Autodesk Fusion 360 part; units mm, degrees
(part 3 of 5)
  spline S11 degree 5 poles (-26.6259, 4.9636) (-26.6188, 4.9697) (-26.6047, 4.9821) (-26.5837, 5.0007) (-26.5558, 5.0255) (-26.5211, 5.0567) (-26.4867, 5.0881) (-26.4526, 5.1196) (-26.4187, 5.1512) (-26.385, 5.183) (-26.3516, 5.2149) (-26.3185, 5.2469) (-26.2856, 5.2791) (-26.2529, 5.3114) (-26.2205, 5.3438) (-26.1884, 5.3764) (-26.1566, 5.4091) (-26.125, 5.4419) (-26.0937, 5.4749) (-26.0626, 5.5079) (-26.0318, 5.5412) (-26.0013, 5.5745) (-25.9711, 5.608) (-25.9412, 5.6416) (-25.9115, 5.6753) (-25.8821, 5.7092) (-25.853, 5.7432) (-25.8242, 5.7773) (-25.7957, 5.8115) (-25.7675, 5.8458) (-25.7396, 5.8803) (-25.712, 5.9149) (-25.6847, 5.9496) (-25.6577, 5.9845) (-25.631, 6.0194) (-25.6046, 6.0545) (-25.5785, 6.0897) (-25.5528, 6.125) (-25.5273, 6.1604) (-25.5022, 6.196) (-25.4775, 6.2316) (-25.453, 6.2674) (-25.4289, 6.3033) (-25.4052, 6.3393) (-25.3818, 6.3754) (-25.3588, 6.4117) (-25.3361, 6.448) (-25.3138, 6.4845) (-25.2919, 6.521) (-25.2703, 6.5577) (-25.2491, 6.5945) (-25.2283, 6.6314) (-25.208, 6.6684) (-25.1881, 6.7055) (-25.1686, 6.7428) (-25.1495, 6.7801) (-25.1308, 6.8176) (-25.1125, 6.8552) (-25.0946, 6.8928) (-25.0772, 6.9306) (-25.0603, 6.9685) (-25.044, 7.0065) (-25.0285, 7.0447) (-25.0136, 7.083) (-24.9994, 7.1214) (-24.9856, 7.16) (-24.9721, 7.1986) (-24.959, 7.2372) (-24.9464, 7.2759) (-24.9347, 7.3148) (-24.9243, 7.3539) (-24.9176, 7.3854) (-24.9137, 7.4093) (-24.9115, 7.4253) (-24.9106, 7.4333) knots -1 -1 -1 -1 -1 -1 -0.98571429 -0.97142857 -0.95714286 -0.94285714 -0.92857143 -0.91428571 -0.9 -0.88571429 -0.87142857 -0.85714286 -0.84285714 -0.82857143 -0.81428571 -0.8 -0.78571429 -0.77142857 -0.75714286 -0.74285714 -0.72857143 -0.71428571 -0.7 -0.68571429 -0.67142857 -0.65714286 -0.64285714 -0.62857143 -0.61428571 -0.6 -0.58571429 -0.57142857 -0.55714286 -0.54285714 -0.52857143 -0.51428571 -0.5 -0.48571429 -0.47142857 -0.45714286 -0.44285714 -0.42857143 -0.41428571 -0.4 -0.38571429 -0.37142857 -0.35714286 -0.34285714 -0.32857143 -0.31428571 -0.3 -0.28571429 -0.27142857 -0.25714286 -0.24285714 -0.22857143 -0.21428571 -0.2 -0.18571429 -0.17142857 -0.15714286 -0.14285714 -0.12857143 -0.11428571 -0.1 -0.08571429 -0.07142857 -0.05714286 -0.04285714 -0.02857143 -0.01428571 0 0 0 0 0 0
  line L11 (-24.9106, 7.4333) -> (-24.8202, 8.2036)
  arc A23 (-23.806, 9.0868) -> (-24.8202, 8.2036) centre (-23.827, 8.087) ccw
  arc A24 (-23.806, 9.0868) -> (-23.405, 9.0868) centre (-23.6055, 18.6339) ccw
  arc A25 (-22.3908, 8.2036) -> (-23.405, 9.0868) centre (-23.384, 8.087) ccw
  line L12 (-22.3908, 8.2036) -> (-22.3005, 7.4333)
  spline S12 degree 5 poles (-22.3005, 7.4333) (-22.2995, 7.4253) (-22.2974, 7.4093) (-22.2934, 7.3854) (-22.2867, 7.3539) (-22.2764, 7.3148) (-22.2646, 7.2759) (-22.252, 7.2372) (-22.2389, 7.1986) (-22.2255, 7.16) (-22.2117, 7.1214) (-22.1974, 7.083) (-22.1825, 7.0447) (-22.167, 7.0065) (-22.1507, 6.9685) (-22.1339, 6.9306) (-22.1164, 6.8928) (-22.0985, 6.8552) (-22.0802, 6.8176) (-22.0615, 6.7801) (-22.0425, 6.7428) (-22.023, 6.7055) (-22.0031, 6.6684) (-21.9827, 6.6314) (-21.962, 6.5945) (-21.9408, 6.5577) (-21.9192, 6.521) (-21.8972, 6.4845) (-21.8749, 6.448) (-21.8522, 6.4117) (-21.8292, 6.3754) (-21.8058, 6.3393) (-21.7821, 6.3033) (-21.758, 6.2674) (-21.7336, 6.2316) (-21.7088, 6.196) (-21.6837, 6.1604) (-21.6583, 6.125) (-21.6325, 6.0897) (-21.6065, 6.0545) (-21.5801, 6.0194) (-21.5534, 5.9845) (-21.5264, 5.9496) (-21.4991, 5.9149) (-21.4714, 5.8803) (-21.4435, 5.8458) (-21.4153, 5.8115) (-21.3868, 5.7773) (-21.358, 5.7432) (-21.3289, 5.7092) (-21.2995, 5.6753) (-21.2699, 5.6416) (-21.2399, 5.608) (-21.2097, 5.5745) (-21.1792, 5.5412) (-21.1484, 5.5079) (-21.1174, 5.4749) (-21.0861, 5.4419) (-21.0545, 5.4091) (-21.0226, 5.3764) (-20.9905, 5.3438) (-20.9581, 5.3114) (-20.9255, 5.2791) (-20.8926, 5.2469) (-20.8594, 5.2149) (-20.826, 5.183) (-20.7924, 5.1512) (-20.7585, 5.1196) (-20.7243, 5.0881) (-20.6899, 5.0567) (-20.6553, 5.0255) (-20.6273, 5.0007) (-20.6063, 4.9821) (-20.5922, 4.9697) (-20.5852, 4.9636) knots 0 0 0 0 0 0 0.01428571 0.02857143 0.04285714 0.05714286 0.07142857 0.08571429 0.1 0.11428571 0.12857143 0.14285714 0.15714286 0.17142857 0.18571429 0.2 0.21428571 0.22857143 0.24285714 0.25714286 0.27142857 0.28571429 0.3 0.31428571 0.32857143 0.34285714 0.35714286 0.37142857 0.38571429 0.4 0.41428571 0.42857143 0.44285714 0.45714286 0.47142857 0.48571429 0.5 0.51428571 0.52857143 0.54285714 0.55714286 0.57142857 0.58571429 0.6 0.61428571 0.62857143 0.64285714 0.65714286 0.67142857 0.68571429 0.7 0.71428571 0.72857143 0.74285714 0.75714286 0.77142857 0.78571429 0.8 0.81428571 0.82857143 0.84285714 0.85714286 0.87142857 0.88571429 0.9 0.91428571 0.92857143 0.94285714 0.95714286 0.97142857 0.98571429 1 1 1 1 1 1
  arc A26 (-20.5852, 4.9636) -> (-19.3861, 5.2849) centre (-23.6055, 18.6339) ccw
  spline S13 degree 5 poles (-19.3861, 5.2849) (-19.383, 5.2937) (-19.377, 5.3115) (-19.3681, 5.3381) (-19.3564, 5.3736) (-19.3419, 5.4179) (-19.3278, 5.4623) (-19.314, 5.5066) (-19.3004, 5.551) (-19.2872, 5.5953) (-19.2742, 5.6396) (-19.2615, 5.6839) (-19.2491, 5.7282) (-19.237, 5.7725) (-19.2252, 5.8168) (-19.2136, 5.8611) (-19.2024, 5.9053) (-19.1915, 5.9496) (-19.1808, 5.9938) (-19.1705, 6.0379) (-19.1604, 6.0821) (-19.1507, 6.1262) (-19.1413, 6.1703) (-19.1321, 6.2144) (-19.1233, 6.2584) (-19.1148, 6.3025) (-19.1066, 6.3464) (-19.0987, 6.3904) (-19.0911, 6.4343) (-19.0838, 6.4781) (-19.0769, 6.5219) (-19.0703, 6.5657) (-19.064, 6.6094) (-19.058, 6.6531) (-19.0524, 6.6967) (-19.0471, 6.7403) (-19.0421, 6.7838) (-19.0374, 6.8273) (-19.0331, 6.8706) (-19.0292, 6.914) (-19.0255, 6.9572) (-19.0223, 7.0004) (-19.0194, 7.0436) (-19.0168, 7.0866) (-19.0146, 7.1296) (-19.0128, 7.1725) (-19.0113, 7.2153) (-19.0102, 7.258) (-19.0095, 7.3007) (-19.0091, 7.3432) (-19.0092, 7.3857) (-19.0096, 7.428) (-19.0105, 7.4703) (-19.0119, 7.5124) (-19.0136, 7.5544) (-19.0158, 7.5963) (-19.0183, 7.638) (-19.0213, 7.6797) (-19.0246, 7.7213) (-19.0284, 7.7627) (-19.0327, 7.8039) (-19.0376, 7.845) (-19.0432, 7.8858) (-19.0495, 7.9265) (-19.0564, 7.9669) (-19.0637, 8.0071) (-19.0714, 8.0473) (-19.0794, 8.0873) (-19.0878, 8.1271) (-19.097, 8.1667) (-19.1076, 8.2057) (-19.1176, 8.2364) (-19.1261, 8.259) (-19.1323, 8.274) (-19.1355, 8.2814) knots -1 -1 -1 -1 -1 -1 -0.98571429 -0.97142857 -0.95714286 -0.94285714 -0.92857143 -0.91428571 -0.9 -0.88571429 -0.87142857 -0.85714286 -0.84285714 -0.82857143 -0.81428571 -0.8 -0.78571429 -0.77142857 -0.75714286 -0.74285714 -0.72857143 -0.71428571 -0.7 -0.68571429 -0.67142857 -0.65714286 -0.64285714 -0.62857143 -0.61428571 -0.6 -0.58571429 -0.57142857 -0.55714286 -0.54285714 -0.52857143 -0.51428571 -0.5 -0.48571429 -0.47142857 -0.45714286 -0.44285714 -0.42857143 -0.41428571 -0.4 -0.38571429 -0.37142857 -0.35714286 -0.34285714 -0.32857143 -0.31428571 -0.3 -0.28571429 -0.27142857 -0.25714286 -0.24285714 -0.22857143 -0.21428571 -0.2 -0.18571429 -0.17142857 -0.15714286 -0.14285714 -0.12857143 -0.11428571 -0.1 -0.08571429 -0.07142857 -0.05714286 -0.04285714 -0.02857143 -0.01428571 0 0 0 0 0 0
  line L13 (-19.1355, 8.2814) -> (-19.4423, 8.9936)
  arc A27 (-19.0056, 10.2656) -> (-19.4423, 8.9936) centre (-18.5239, 9.3893) ccw
  circle A28 centre (-23.6055, 18.6339) radius 2.5
  line L14 (-23.6055, 18.6339) -> (1.0147, 14.2927)
  line L15 (-23.6055, 18.6339) -> (1.3945, 18.6339) construction
  line L16 (-23.6055, 18.6339) -> (1.0147, 22.9751)
  line L17 (-23.6055, 18.6339) -> (1.3945, 18.6339) construction
  circle A29 centre (1.3945, 18.6339) radius 4.3578
  circle A30 centre (-23.6055, 18.6339) radius 9.5492
  circle A31 centre (1.3945, 18.6339) radius 2
  dimension "d11" = 25
  dimension "d12" = 10
  dimension "d13" = 25
  dimension "d14" = 10
  dimension "d15" = 4
  constraint horizontal L15
  constraint coincident A0.centre A2.centre
  constraint horizontal L17
  constraint coincident L15.end L17.end
  constraint coincident L16.end A29
  constraint concentric A29 A31
  measures "d11" distance of A0.centre L14.end
  measures "d12" angle of L14 L15
  measures "d13" distance of A0.centre L16.end
  measures "d14" angle of L16 L17
  measures "d15" diameter of A31
extrude "Extrude4" add sketch "Sketch2 (2)" against normal blind 5 contours A0 L14 L16 A29 A30 | L14 L16 A29 sketch seen with x (0.937437, -0.333603, -0.099601) y (0.345241, 0.927672, 0.142244) z (0.044943, -0.167731, 0.984808) at (-27.624, 11.8894, -48.8944) in component "Spur Gear (12 teeth)"
fillet "Fillet2" radius 5 2 edges at (-8.6545, -4.0357, 2.5) (-9.5129, -0.8323, 2.5) in component "Spur Gear (12 teeth)"
component "Spur Gear (12 teeth)" placed x (1, 0, 0) y (0, 1, 0) z (0, 0, 1) at (0, 0, 0)

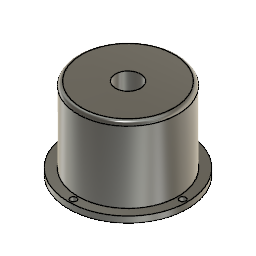
design "Base"
Autodesk Fusion 360 part; units mm, degrees
sketch "Sketch1" plane through (0, 0, 0) normal (0, 0, 1) x (1, 0, 0)
  circle A0 centre (0, 0) radius 10
  circle A1 centre (0, 0) radius 47.5
  circle A2 centre (-43.75, 0) radius 2.5
  line L0 (0, 0) -> (-43.75, 0) construction
  circle A3 centre (0, -43.75) radius 2.5
  circle A4 centre (43.75, 0) radius 2.5
  circle A5 centre (0, 43.75) radius 2.5
  circle A6 centre (0, 0) radius 32.5 construction
  circle A7 centre (0, 0) radius 40
  dimension "d1" = 20
  dimension "d2" = 95
  dimension "d3" = 5
  dimension "d4" = 43.75
  dimension "d6" = 360
  dimension "d7" = 65
  dimension "d16" = 80
  constraint coincident A0.centre A1.centre
  constraint coincident A2.centre L0.end
  constraint horizontal L0
  measures "d1" diameter of A0
  measures "d2" diameter of A1
  measures "d3" diameter of A2
  measures "d4" distance of A0.centre A2.centre
  measures "d7" diameter of A6
  measures "d16" diameter of A7
extrude "Extrude1" add sketch "Sketch1" along normal blind 5 contours A1 | A7
extrude "Extrude2" add sketch "Sketch1" along normal blind 60 thin wall 7.5 inside contours A7
sketch "Sketch2" plane through (0, 0, 60) normal (0, 0, 1) x (-1, 0, 0)
  circle A0 centre (0, 0) radius 10
  circle A1 centre (0, 0) radius 40
extrude "Extrude3" add sketch "Sketch2" along normal blind 5
ref_plane "WorkPlane1" through (0, 0, 55) normal (0, 0, 1) x (-1, 0, 0)
sketch "Sketch3" plane through (0, 0, 55) normal (0, 0, 1) x (1, 0, 0)
  circle A0 centre (0, 0) radius 32.5
  circle A1 centre (0, 0) radius 17.5
  line L0 (2.5, -32.4037) -> (2.5, -17.3205)
  line L1 (2.5, 17.3205) -> (2.5, 32.4037)
  line L2 (-17.3205, 2.5) -> (-32.4037, 2.5)
  line L3 (-2.5, -32.4037) -> (-2.5, -17.3205)
  line L4 (17.3205, 2.5) -> (32.4037, 2.5)
  line L5 (-2.5, 17.3205) -> (-2.5, 32.4037)
  line L6 (-17.3205, -2.5) -> (-32.4037, -2.5)
  line L7 (17.3205, -2.5) -> (32.4037, -2.5)
  constraint coincident A0 L0.start
  constraint coincident A0 L3.start
  constraint coincident A1 L0.end
  constraint coincident A1 L3.end
  constraint coincident A1 L6.start
  constraint coincident A1 L2.start
  constraint coincident A1 L5.start
  constraint coincident A1 L1.start
  constraint coincident A1 L4.start
  constraint coincident A0 L4.end
  constraint coincident A0 L5.end
  constraint coincident A0 L1.end
  constraint coincident A0 L7.end
  constraint coincident A1 L7.start
  constraint coincident A0 L2.end
  constraint coincident A0 L6.end
extrude "Extrude4" cut sketch "Sketch3" along normal blind 5 and the other way through all contours A0 A1 L1 L4 | A0 A1 L0 L7 | A0 A1 L2 L5 | A0 A1 L3 L6
fillet "Fillet1" radius 3 1 edges at (37.2931, 14.4646, 65)
equation "Thickness = 15 mm"
equation "d9 = Thickness / 3"
equation "d11 = Thickness / 2"
equation "d12 = Thickness * 4"
equation "d14 = Thickness / 3"

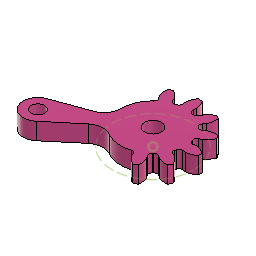
design "Spur Gear-Right"
description: Spur Gear; Module: 2.0; Num Teeth: 12; Pressure Angle: 20.0; Backlash: 0.00 mm
Autodesk Fusion 360 part; units mm, degrees
derive "DerivedContext1" from "Assembly v8"
sketch "Sketch1" plane through (0, 0, 0) normal (0, 0, 1) x (1, 0, 0) in component "Spur Gear (12 teeth)"
  circle A0 centre (0, 0) radius 9.5492
  circle A1 centre (0, 0) radius 2.5
extrude "Extrude1" add sketch "Sketch1" along normal blind 5 in component "Spur Gear (12 teeth)"
sketch "Sketch2" plane through (0, 0, 0) normal (0, 0, 1) x (1, 0, 0) in component "Spur Gear (12 teeth)"
  spline S0 degree 5 poles (11.1567, -1.6383) (11.1647, -1.6395) (11.1807, -1.6416) (11.2048, -1.6439) (11.237, -1.6456) (11.2774, -1.6458) (11.318, -1.6445) (11.3587, -1.6423) (11.3994, -1.6396) (11.4401, -1.6366) (11.4809, -1.6333) (11.5218, -1.6295) (11.5626, -1.625) (11.6035, -1.6199) (11.6445, -1.614) (11.6854, -1.6075) (11.7264, -1.6005) (11.7674, -1.5929) (11.8084, -1.585) (11.8494, -1.5766) (11.8905, -1.5678) (11.9315, -1.5587) (11.9725, -1.5491) (12.0135, -1.539) (12.0545, -1.5285) (12.0956, -1.5175) (12.1366, -1.5062) (12.1776, -1.4944) (12.2186, -1.4823) (12.2595, -1.4698) (12.3005, -1.4569) (12.3414, -1.4437) (12.3824, -1.4301) (12.4233, -1.4161) (12.4641, -1.4018) (12.505, -1.3871) (12.5458, -1.372) (12.5866, -1.3566) (12.6274, -1.3409) (12.6681, -1.3248) (12.7088, -1.3084) (12.7495, -1.2917) (12.7902, -1.2746) (12.8308, -1.2572) (12.8713, -1.2395) (12.9119, -1.2215) (12.9523, -1.2031) (12.9928, -1.1844) (13.0332, -1.1654) (13.0735, -1.1461) (13.1138, -1.1265) (13.1541, -1.1066) (13.1943, -1.0863) (13.2345, -1.0658) (13.2746, -1.045) (13.3146, -1.0239) (13.3546, -1.0024) (13.3946, -0.9807) (13.4344, -0.9587) (13.4743, -0.9364) (13.514, -0.9138) (13.5538, -0.8909) (13.5934, -0.8678) (13.633, -0.8443) (13.6725, -0.8206) (13.712, -0.7966) (13.7514, -0.7723) (13.7907, -0.7477) (13.8299, -0.7229) (13.8691, -0.6978) (13.9082, -0.6724) (13.9395, -0.6518) (13.9629, -0.6363) (13.9784, -0.6259) (13.9862, -0.6207) knots 0 0 0 0 0 0 0.01428571 0.02857143 0.04285714 0.05714286 0.07142857 0.08571429 0.1 0.11428571 0.12857143 0.14285714 0.15714286 0.17142857 0.18571429 0.2 0.21428571 0.22857143 0.24285714 0.25714286 0.27142857 0.28571429 0.3 0.31428571 0.32857143 0.34285714 0.35714286 0.37142857 0.38571429 0.4 0.41428571 0.42857143 0.44285714 0.45714286 0.47142857 0.48571429 0.5 0.51428571 0.52857143 0.54285714 0.55714286 0.57142857 0.58571429 0.6 0.61428571 0.62857143 0.64285714 0.65714286 0.67142857 0.68571429 0.7 0.71428571 0.72857143 0.74285714 0.75714286 0.77142857 0.78571429 0.8 0.81428571 0.82857143 0.84285714 0.85714286 0.87142857 0.88571429 0.9 0.91428571 0.92857143 0.94285714 0.95714286 0.97142857 0.98571429 1 1 1 1 1 1
  spline S1 degree 5 poles (11.1567, 1.6383) (11.1647, 1.6395) (11.1807, 1.6416) (11.2048, 1.6439) (11.237, 1.6456) (11.2774, 1.6458) (11.318, 1.6445) (11.3587, 1.6423) (11.3994, 1.6396) (11.4401, 1.6366) (11.4809, 1.6333) (11.5218, 1.6295) (11.5626, 1.625) (11.6035, 1.6199) (11.6445, 1.614) (11.6854, 1.6075) (11.7264, 1.6005) (11.7674, 1.5929) (11.8084, 1.585) (11.8494, 1.5766) (11.8905, 1.5678) (11.9315, 1.5587) (11.9725, 1.5491) (12.0135, 1.539) (12.0545, 1.5285) (12.0956, 1.5175) (12.1366, 1.5062) (12.1776, 1.4944) (12.2186, 1.4823) (12.2595, 1.4698) (12.3005, 1.4569) (12.3414, 1.4437) (12.3824, 1.4301) (12.4233, 1.4161) (12.4641, 1.4018) (12.505, 1.3871) (12.5458, 1.372) (12.5866, 1.3566) (12.6274, 1.3409) (12.6681, 1.3248) (12.7088, 1.3084) (12.7495, 1.2917) (12.7902, 1.2746) (12.8308, 1.2572) (12.8713, 1.2395) (12.9119, 1.2215) (12.9523, 1.2031) (12.9928, 1.1844) (13.0332, 1.1654) (13.0735, 1.1461) (13.1138, 1.1265) (13.1541, 1.1066) (13.1943, 1.0863) (13.2345, 1.0658) (13.2746, 1.045) (13.3146, 1.0239) (13.3546, 1.0024) (13.3946, 0.9807) (13.4344, 0.9587) (13.4743, 0.9364) (13.514, 0.9138) (13.5538, 0.8909) (13.5934, 0.8678) (13.633, 0.8443) (13.6725, 0.8206) (13.712, 0.7966) (13.7514, 0.7723) (13.7907, 0.7477) (13.8299, 0.7229) (13.8691, 0.6978) (13.9082, 0.6724) (13.9395, 0.6518) (13.9629, 0.6363) (13.9784, 0.6259) (13.9862, 0.6207) knots 0 0 0 0 0 0 0.01428571 0.02857143 0.04285714 0.05714286 0.07142857 0.08571429 0.1 0.11428571 0.12857143 0.14285714 0.15714286 0.17142857 0.18571429 0.2 0.21428571 0.22857143 0.24285714 0.25714286 0.27142857 0.28571429 0.3 0.31428571 0.32857143 0.34285714 0.35714286 0.37142857 0.38571429 0.4 0.41428571 0.42857143 0.44285714 0.45714286 0.47142857 0.48571429 0.5 0.51428571 0.52857143 0.54285714 0.55714286 0.57142857 0.58571429 0.6 0.61428571 0.62857143 0.64285714 0.65714286 0.67142857 0.68571429 0.7 0.71428571 0.72857143 0.74285714 0.75714286 0.77142857 0.78571429 0.8 0.81428571 0.82857143 0.84285714 0.85714286 0.87142857 0.88571429 0.9 0.91428571 0.92857143 0.94285714 0.95714286 0.97142857 0.98571429 1 1 1 1 1 1
  arc A0 (13.9862, -0.6207) -> (13.9862, 0.6207) centre (0, 0) ccw
  line L0 (9.438, -1.3874) -> (11.1567, -1.6383)
  line L1 (9.438, 1.3874) -> (11.1567, 1.6383)
  line L2 (9.438, -1.3874) -> (9.438, 1.3874)
  point P0 (11.3527, -1.6425)
  point P1 (11.5515, -1.6261)
  point P2 (11.7521, -1.5957)
  point P3 (11.954, -1.5533)
  point P4 (12.1568, -1.5003)
  point P5 (12.3603, -1.4374)
  point P6 (12.5642, -1.3651)
  point P7 (12.7683, -1.2838)
  point P8 (12.9724, -1.1938)
  point P9 (13.1764, -1.0953)
  point P10 (13.3799, -0.9887)
  point P11 (13.5828, -0.8739)
  point P12 (13.785, -0.7512)
  point P13 (11.3527, 1.6425)
  point P14 (11.5515, 1.6261)
  point P15 (11.7521, 1.5957)
  point P16 (11.954, 1.5533)
  point P17 (12.1568, 1.5003)
  point P18 (12.3603, 1.4374)
  point P19 (12.5642, 1.3651)
  point P20 (12.7683, 1.2838)
  point P21 (12.9724, 1.1938)
  point P22 (13.1764, 1.0953)
  point P23 (13.3799, 0.9887)
  point P24 (13.5828, 0.8739)
  point P25 (13.785, 0.7512)
extrude "Extrude2" add sketch "Sketch2" along normal blind 5 in component "Spur Gear (12 teeth)"
fillet "Fillet1" radius 1 2 edges at (9.4477, -1.3888, 2.5) (9.4477, 1.3888, 2.5) in component "Spur Gear (12 teeth)"
pattern_circular "C-Pattern1" count 12 over 360 about axis through (0, 0, 0) along (0, 0, 1) of "Extrude2", "Fillet1" in component "Spur Gear (12 teeth)"
sketch "Sketch3" plane through (0, 0, 0) normal (0, 0, 1) x (1, 0, 0) in component "Spur Gear (12 teeth)"
  circle A0 centre (0, 0) radius 12 construction
sketch "Sketch1 (2)" plane through (0, 0, 5) normal (0, 0, 1) x (-1, 0, 0)
  arc A0 (-9.1699, 2.6646) -> (-9.2737, 2.2773) centre (0, 0) ccw
  arc A1 (-10.3893, 1.5263) -> (-9.2737, 2.2773) centre (-10.2448, 2.5158) ccw
  line L0 (-10.3893, 1.5263) -> (-11.1567, 1.6383)
  spline S0 degree 5 poles (-11.1567, 1.6383) (-11.1647, 1.6395) (-11.1807, 1.6416) (-11.2048, 1.6439) (-11.237, 1.6456) (-11.2774, 1.6458) (-11.318, 1.6445) (-11.3587, 1.6423) (-11.3994, 1.6396) (-11.4401, 1.6366) (-11.4809, 1.6333) (-11.5218, 1.6295) (-11.5626, 1.625) (-11.6035, 1.6199) (-11.6445, 1.614) (-11.6854, 1.6075) (-11.7264, 1.6005) (-11.7674, 1.5929) (-11.8084, 1.585) (-11.8494, 1.5766) (-11.8905, 1.5678) (-11.9315, 1.5587) (-11.9725, 1.5491) (-12.0135, 1.539) (-12.0545, 1.5285) (-12.0956, 1.5175) (-12.1366, 1.5062) (-12.1776, 1.4944) (-12.2186, 1.4823) (-12.2595, 1.4698) (-12.3005, 1.4569) (-12.3414, 1.4437) (-12.3824, 1.4301) (-12.4233, 1.4161) (-12.4641, 1.4018) (-12.505, 1.3871) (-12.5458, 1.372) (-12.5866, 1.3566) (-12.6274, 1.3409) (-12.6681, 1.3248) (-12.7088, 1.3084) (-12.7495, 1.2917) (-12.7902, 1.2746) (-12.8308, 1.2572) (-12.8713, 1.2395) (-12.9119, 1.2215) (-12.9523, 1.2031) (-12.9928, 1.1844) (-13.0332, 1.1654) (-13.0735, 1.1461) (-13.1138, 1.1265) (-13.1541, 1.1066) (-13.1943, 1.0863) (-13.2345, 1.0658) (-13.2746, 1.045) (-13.3146, 1.0239) (-13.3546, 1.0024) (-13.3946, 0.9807) (-13.4344, 0.9587) (-13.4743, 0.9364) (-13.514, 0.9138) (-13.5538, 0.8909) (-13.5934, 0.8678) (-13.633, 0.8443) (-13.6725, 0.8206) (-13.712, 0.7966) (-13.7514, 0.7723) (-13.7907, 0.7477) (-13.8299, 0.7229) (-13.8691, 0.6978) (-13.9082, 0.6724) (-13.9395, 0.6518) (-13.9629, 0.6363) (-13.9784, 0.6259) (-13.9862, 0.6207) knots 0 0 0 0 0 0 0.01428571 0.02857143 0.04285714 0.05714286 0.07142857 0.08571429 0.1 0.11428571 0.12857143 0.14285714 0.15714286 0.17142857 0.18571429 0.2 0.21428571 0.22857143 0.24285714 0.25714286 0.27142857 0.28571429 0.3 0.31428571 0.32857143 0.34285714 0.35714286 0.37142857 0.38571429 0.4 0.41428571 0.42857143 0.44285714 0.45714286 0.47142857 0.48571429 0.5 0.51428571 0.52857143 0.54285714 0.55714286 0.57142857 0.58571429 0.6 0.61428571 0.62857143 0.64285714 0.65714286 0.67142857 0.68571429 0.7 0.71428571 0.72857143 0.74285714 0.75714286 0.77142857 0.78571429 0.8 0.81428571 0.82857143 0.84285714 0.85714286 0.87142857 0.88571429 0.9 0.91428571 0.92857143 0.94285714 0.95714286 0.97142857 0.98571429 1 1 1 1 1 1
  arc A2 (-13.9862, 0.6207) -> (-13.9862, -0.6207) centre (0, 0) ccw
  spline S1 degree 5 poles (-13.9862, -0.6207) (-13.9784, -0.6259) (-13.9629, -0.6363) (-13.9395, -0.6518) (-13.9082, -0.6724) (-13.8691, -0.6978) (-13.8299, -0.7229) (-13.7907, -0.7477) (-13.7514, -0.7723) (-13.712, -0.7966) (-13.6725, -0.8206) (-13.633, -0.8443) (-13.5934, -0.8678) (-13.5538, -0.8909) (-13.514, -0.9138) (-13.4743, -0.9364) (-13.4344, -0.9587) (-13.3946, -0.9807) (-13.3546, -1.0024) (-13.3146, -1.0239) (-13.2746, -1.045) (-13.2345, -1.0658) (-13.1943, -1.0863) (-13.1541, -1.1066) (-13.1138, -1.1265) (-13.0735, -1.1461) (-13.0332, -1.1654) (-12.9928, -1.1844) (-12.9523, -1.2031) (-12.9119, -1.2215) (-12.8713, -1.2395) (-12.8308, -1.2572) (-12.7902, -1.2746) (-12.7495, -1.2917) (-12.7088, -1.3084) (-12.6681, -1.3248) (-12.6274, -1.3409) (-12.5866, -1.3566) (-12.5458, -1.372) (-12.505, -1.3871) (-12.4641, -1.4018) (-12.4233, -1.4161) (-12.3824, -1.4301) (-12.3414, -1.4437) (-12.3005, -1.4569) (-12.2595, -1.4698) (-12.2186, -1.4823) (-12.1776, -1.4944) (-12.1366, -1.5062) (-12.0956, -1.5175) (-12.0545, -1.5285) (-12.0135, -1.539) (-11.9725, -1.5491) (-11.9315, -1.5587) (-11.8905, -1.5678) (-11.8494, -1.5766) (-11.8084, -1.585) (-11.7674, -1.5929) (-11.7264, -1.6005) (-11.6854, -1.6075) (-11.6445, -1.614) (-11.6035, -1.6199) (-11.5626, -1.625) (-11.5218, -1.6295) (-11.4809, -1.6333) (-11.4401, -1.6366) (-11.3994, -1.6396) (-11.3587, -1.6423) (-11.318, -1.6445) (-11.2774, -1.6458) (-11.237, -1.6456) (-11.2048, -1.6439) (-11.1807, -1.6416) (-11.1647, -1.6395) (-11.1567, -1.6383) knots -1 -1 -1 -1 -1 -1 -0.98571429 -0.97142857 -0.95714286 -0.94285714 -0.92857143 -0.91428571 -0.9 -0.88571429 -0.87142857 -0.85714286 -0.84285714 -0.82857143 -0.81428571 -0.8 -0.78571429 -0.77142857 -0.75714286 -0.74285714 -0.72857143 -0.71428571 -0.7 -0.68571429 -0.67142857 -0.65714286 -0.64285714 -0.62857143 -0.61428571 -0.6 -0.58571429 -0.57142857 -0.55714286 -0.54285714 -0.52857143 -0.51428571 -0.5 -0.48571429 -0.47142857 -0.45714286 -0.44285714 -0.42857143 -0.41428571 -0.4 -0.38571429 -0.37142857 -0.35714286 -0.34285714 -0.32857143 -0.31428571 -0.3 -0.28571429 -0.27142857 -0.25714286 -0.24285714 -0.22857143 -0.21428571 -0.2 -0.18571429 -0.17142857 -0.15714286 -0.14285714 -0.12857143 -0.11428571 -0.1 -0.08571429 -0.07142857 -0.05714286 -0.04285714 -0.02857143 -0.01428571 0 0 0 0 0 0
  line L1 (-11.1567, -1.6383) -> (-10.3893, -1.5263)
  arc A3 (-9.2737, -2.2773) -> (-10.3893, -1.5263) centre (-10.2448, -2.5158) ccw
  arc A4 (-9.2737, -2.2773) -> (-9.1699, -2.6646) centre (0, 0) ccw
  arc A5 (-9.7605, -3.8729) -> (-9.1699, -2.6646) centre (-10.1302, -2.9437) ccw
  line L2 (-9.7605, -3.8729) -> (-10.4811, -4.1595)
  spline S2 degree 5 poles (-10.4811, -4.1595) (-10.4886, -4.1625) (-10.5035, -4.1687) (-10.5256, -4.1787) (-10.5543, -4.1933) (-10.5894, -4.2134) (-10.6239, -4.2349) (-10.658, -4.2571) (-10.692, -4.2797) (-10.7258, -4.3027) (-10.7594, -4.326) (-10.7929, -4.3497) (-10.826, -4.374) (-10.8589, -4.3989) (-10.8914, -4.4244) (-10.9236, -4.4505) (-10.9556, -4.4772) (-10.9873, -4.5042) (-11.0189, -4.5316) (-11.0502, -4.5593) (-11.0814, -4.5874) (-11.1123, -4.6159) (-11.143, -4.6447) (-11.1735, -4.674) (-11.2038, -4.7036) (-11.2338, -4.7336) (-11.2637, -4.7639) (-11.2933, -4.7946) (-11.3227, -4.8256) (-11.352, -4.8569) (-11.381, -4.8885) (-11.4099, -4.9204) (-11.4385, -4.9527) (-11.4669, -4.9852) (-11.4952, -5.0181) (-11.5232, -5.0512) (-11.551, -5.0847) (-11.5787, -5.1184) (-11.6061, -5.1524) (-11.6334, -5.1867) (-11.6604, -5.2213) (-11.6873, -5.2561) (-11.7139, -5.2912) (-11.7404, -5.3266) (-11.7666, -5.3622) (-11.7927, -5.3981) (-11.8186, -5.4343) (-11.8443, -5.4707) (-11.8698, -5.5073) (-11.8951, -5.5442) (-11.9202, -5.5813) (-11.9451, -5.6187) (-11.9698, -5.6563) (-11.9943, -5.6942) (-12.0186, -5.7323) (-12.0427, -5.7706) (-12.0667, -5.8092) (-12.0904, -5.848) (-12.1139, -5.887) (-12.1373, -5.9262) (-12.1604, -5.9656) (-12.1834, -6.0053) (-12.2061, -6.0452) (-12.2287, -6.0853) (-12.251, -6.1256) (-12.2732, -6.1661) (-12.2952, -6.2069) (-12.3169, -6.2478) (-12.3385, -6.2889) (-12.3599, -6.3303) (-12.3811, -6.3718) (-12.3979, -6.4052) (-12.4104, -6.4304) (-12.4186, -6.4472) (-12.4228, -6.4556) knots 0 0 0 0 0 0 0.01428571 0.02857143 0.04285714 0.05714286 0.07142857 0.08571429 0.1 0.11428571 0.12857143 0.14285714 0.15714286 0.17142857 0.18571429 0.2 0.21428571 0.22857143 0.24285714 0.25714286 0.27142857 0.28571429 0.3 0.31428571 0.32857143 0.34285714 0.35714286 0.37142857 0.38571429 0.4 0.41428571 0.42857143 0.44285714 0.45714286 0.47142857 0.48571429 0.5 0.51428571 0.52857143 0.54285714 0.55714286 0.57142857 0.58571429 0.6 0.61428571 0.62857143 0.64285714 0.65714286 0.67142857 0.68571429 0.7 0.71428571 0.72857143 0.74285714 0.75714286 0.77142857 0.78571429 0.8 0.81428571 0.82857143 0.84285714 0.85714286 0.87142857 0.88571429 0.9 0.91428571 0.92857143 0.94285714 0.95714286 0.97142857 0.98571429 1 1 1 1 1 1
  arc A6 (-12.4228, -6.4556) -> (-11.8021, -7.5307) centre (0, 0) ccw
  spline S3 degree 5 poles (-11.8021, -7.5307) (-11.7927, -7.5313) (-11.774, -7.5325) (-11.746, -7.5342) (-11.7087, -7.5364) (-11.6621, -7.5388) (-11.6156, -7.541) (-11.5692, -7.5429) (-11.5229, -7.5445) (-11.4766, -7.5458) (-11.4305, -7.5469) (-11.3844, -7.5477) (-11.3384, -7.5482) (-11.2924, -7.5484) (-11.2466, -7.5484) (-11.2009, -7.5481) (-11.1552, -7.5475) (-11.1097, -7.5466) (-11.0642, -7.5454) (-11.0189, -7.544) (-10.9736, -7.5423) (-10.9285, -7.5403) (-10.8834, -7.538) (-10.8385, -7.5354) (-10.7937, -7.5325) (-10.7489, -7.5293) (-10.7044, -7.5259) (-10.6599, -7.5221) (-10.6155, -7.5181) (-10.5713, -7.5137) (-10.5271, -7.5091) (-10.4832, -7.5042) (-10.4393, -7.4989) (-10.3956, -7.4934) (-10.352, -7.4876) (-10.3085, -7.4814) (-10.2652, -7.475) (-10.222, -7.4682) (-10.179, -7.4611) (-10.1361, -7.4538) (-10.0934, -7.4461) (-10.0508, -7.438) (-10.0084, -7.4297) (-9.9662, -7.421) (-9.9241, -7.412) (-9.8822, -7.4027) (-9.8404, -7.393) (-9.7989, -7.383) (-9.7575, -7.3727) (-9.7163, -7.362) (-9.6753, -7.351) (-9.6345, -7.3396) (-9.594, -7.3278) (-9.5536, -7.3156) (-9.5135, -7.303) (-9.4736, -7.2901) (-9.4339, -7.2768) (-9.3944, -7.2632) (-9.3551, -7.2492) (-9.3161, -7.2349) (-9.2774, -7.22) (-9.239, -7.2046) (-9.201, -7.1886) (-9.1634, -7.172) (-9.1261, -7.1549) (-9.0891, -7.1374) (-9.0523, -7.1196) (-9.0157, -7.1016) (-8.9794, -7.0831) (-8.9437, -7.064) (-8.9087, -7.0436) (-8.8816, -7.0261) (-8.862, -7.012) (-8.8491, -7.0022) (-8.8428, -6.9972) knots -1 -1 -1 -1 -1 -1 -0.98571429 -0.97142857 -0.95714286 -0.94285714 -0.92857143 -0.91428571 -0.9 -0.88571429 -0.87142857 -0.85714286 -0.84285714 -0.82857143 -0.81428571 -0.8 -0.78571429 -0.77142857 -0.75714286 -0.74285714 -0.72857143 -0.71428571 -0.7 -0.68571429 -0.67142857 -0.65714286 -0.64285714 -0.62857143 -0.61428571 -0.6 -0.58571429 -0.57142857 -0.55714286 -0.54285714 -0.52857143 -0.51428571 -0.5 -0.48571429 -0.47142857 -0.45714286 -0.44285714 -0.42857143 -0.41428571 -0.4 -0.38571429 -0.37142857 -0.35714286 -0.34285714 -0.32857143 -0.31428571 -0.3 -0.28571429 -0.27142857 -0.25714286 -0.24285714 -0.22857143 -0.21428571 -0.2 -0.18571429 -0.17142857 -0.15714286 -0.14285714 -0.12857143 -0.11428571 -0.1 -0.08571429 -0.07142857 -0.05714286 -0.04285714 -0.02857143 -0.01428571 0 0 0 0 0 0
  line L3 (-8.8428, -6.9972) -> (-8.2343, -6.5164)
  arc A7 (-6.8926, -6.609) -> (-8.2343, -6.5164) centre (-7.6144, -7.3011) ccw
  arc A8 (-6.8926, -6.609) -> (-6.609, -6.8926) centre (0, 0) ccw
  arc A9 (-6.5164, -8.2343) -> (-6.609, -6.8926) centre (-7.3011, -7.6144) ccw
  line L4 (-6.5164, -8.2343) -> (-6.9972, -8.8428)
  spline S4 degree 5 poles (-6.9972, -8.8428) (-7.0022, -8.8491) (-7.012, -8.862) (-7.0261, -8.8816) (-7.0436, -8.9087) (-7.064, -8.9437) (-7.0831, -8.9794) (-7.1016, -9.0157) (-7.1196, -9.0523) (-7.1374, -9.0891) (-7.1549, -9.1261) (-7.172, -9.1634) (-7.1886, -9.201) (-7.2046, -9.239) (-7.22, -9.2774) (-7.2349, -9.3161) (-7.2492, -9.3551) (-7.2632, -9.3944) (-7.2768, -9.4339) (-7.2901, -9.4736) (-7.303, -9.5135) (-7.3156, -9.5536) (-7.3278, -9.594) (-7.3396, -9.6345) (-7.351, -9.6753) (-7.362, -9.7163) (-7.3727, -9.7575) (-7.383, -9.7989) (-7.393, -9.8404) (-7.4027, -9.8822) (-7.412, -9.9241) (-7.421, -9.9662) (-7.4297, -10.0084) (-7.438, -10.0508) (-7.4461, -10.0934) (-7.4538, -10.1361) (-7.4611, -10.179) (-7.4682, -10.222) (-7.475, -10.2652) (-7.4814, -10.3085) (-7.4876, -10.352) (-7.4934, -10.3956) (-7.4989, -10.4393) (-7.5042, -10.4832) (-7.5091, -10.5271) (-7.5137, -10.5713) (-7.5181, -10.6155) (-7.5221, -10.6599) (-7.5259, -10.7044) (-7.5293, -10.7489) (-7.5325, -10.7937) (-7.5354, -10.8385) (-7.538, -10.8834) (-7.5403, -10.9285) (-7.5423, -10.9736) (-7.544, -11.0189) (-7.5454, -11.0642) (-7.5466, -11.1097) (-7.5475, -11.1552) (-7.5481, -11.2009) (-7.5484, -11.2466) (-7.5484, -11.2924) (-7.5482, -11.3384) (-7.5477, -11.3844) (-7.5469, -11.4305) (-7.5458, -11.4766) (-7.5445, -11.5229) (-7.5429, -11.5692) (-7.541, -11.6156) (-7.5388, -11.6621) (-7.5364, -11.7087) (-7.5342, -11.746) (-7.5325, -11.774) (-7.5313, -11.7927) (-7.5307, -11.8021) knots 0 0 0 0 0 0 0.01428571 0.02857143 0.04285714 0.05714286 0.07142857 0.08571429 0.1 0.11428571 0.12857143 0.14285714 0.15714286 0.17142857 0.18571429 0.2 0.21428571 0.22857143 0.24285714 0.25714286 0.27142857 0.28571429 0.3 0.31428571 0.32857143 0.34285714 0.35714286 0.37142857 0.38571429 0.4 0.41428571 0.42857143 0.44285714 0.45714286 0.47142857 0.48571429 0.5 0.51428571 0.52857143 0.54285714 0.55714286 0.57142857 0.58571429 0.6 0.61428571 0.62857143 0.64285714 0.65714286 0.67142857 0.68571429 0.7 0.71428571 0.72857143 0.74285714 0.75714286 0.77142857 0.78571429 0.8 0.81428571 0.82857143 0.84285714 0.85714286 0.87142857 0.88571429 0.9 0.91428571 0.92857143 0.94285714 0.95714286 0.97142857 0.98571429 1 1 1 1 1 1
  arc A10 (-7.5307, -11.8021) -> (-6.4556, -12.4228) centre (0, 0) ccw
  spline S5 degree 5 poles (-6.4556, -12.4228) (-6.4472, -12.4186) (-6.4304, -12.4104) (-6.4052, -12.3979) (-6.3718, -12.3811) (-6.3303, -12.3599) (-6.2889, -12.3385) (-6.2478, -12.3169) (-6.2069, -12.2952) (-6.1661, -12.2732) (-6.1256, -12.251) (-6.0853, -12.2287) (-6.0452, -12.2061) (-6.0053, -12.1834) (-5.9656, -12.1604) (-5.9262, -12.1373) (-5.887, -12.1139) (-5.848, -12.0904) (-5.8092, -12.0667) (-5.7706, -12.0427) (-5.7323, -12.0186) (-5.6942, -11.9943) (-5.6563, -11.9698) (-5.6187, -11.9451) (-5.5813, -11.9202) (-5.5442, -11.8951) (-5.5073, -11.8698) (-5.4707, -11.8443) (-5.4343, -11.8186) (-5.3981, -11.7927) (-5.3622, -11.7666) (-5.3266, -11.7404) (-5.2912, -11.7139) (-5.2561, -11.6873) (-5.2213, -11.6604) (-5.1867, -11.6334) (-5.1524, -11.6061) (-5.1184, -11.5787) (-5.0847, -11.551) (-5.0512, -11.5232) (-5.0181, -11.4952) (-4.9852, -11.4669) (-4.9527, -11.4385) (-4.9204, -11.4099) (-4.8885, -11.381) (-4.8569, -11.352) (-4.8256, -11.3227) (-4.7946, -11.2933) (-4.7639, -11.2637) (-4.7336, -11.2338) (-4.7036, -11.2038) (-4.674, -11.1735) (-4.6447, -11.143) (-4.6159, -11.1123) (-4.5874, -11.0814) (-4.5593, -11.0502) (-4.5316, -11.0189) (-4.5042, -10.9873) (-4.4772, -10.9556) (-4.4505, -10.9236) (-4.4244, -10.8914) (-4.3989, -10.8589) (-4.374, -10.826) (-4.3497, -10.7929) (-4.326, -10.7594) (-4.3027, -10.7258) (-4.2797, -10.692) (-4.2571, -10.658) (-4.2349, -10.6239) (-4.2134, -10.5894) (-4.1933, -10.5543) (-4.1787, -10.5256) (-4.1687, -10.5035) (-4.1625, -10.4886) (-4.1595, -10.4811) knots -1 -1 -1 -1 -1 -1 -0.98571429 -0.97142857 -0.95714286 -0.94285714 -0.92857143 -0.91428571 -0.9 -0.88571429 -0.87142857 -0.85714286 -0.84285714 -0.82857143 -0.81428571 -0.8 -0.78571429 -0.77142857 -0.75714286 -0.74285714 -0.72857143 -0.71428571 -0.7 -0.68571429 -0.67142857 -0.65714286 -0.64285714 -0.62857143 -0.61428571 -0.6 -0.58571429 -0.57142857 -0.55714286 -0.54285714 -0.52857143 -0.51428571 -0.5 -0.48571429 -0.47142857 -0.45714286 -0.44285714 -0.42857143 -0.41428571 -0.4 -0.38571429 -0.37142857 -0.35714286 -0.34285714 -0.32857143 -0.31428571 -0.3 -0.28571429 -0.27142857 -0.25714286 -0.24285714 -0.22857143 -0.21428571 -0.2 -0.18571429 -0.17142857 -0.15714286 -0.14285714 -0.12857143 -0.11428571 -0.1 -0.08571429 -0.07142857 -0.05714286 -0.04285714 -0.02857143 -0.01428571 0 0 0 0 0 0
  line L5 (-4.1595, -10.4811) -> (-3.8729, -9.7605)
  arc A11 (-2.6646, -9.1699) -> (-3.8729, -9.7605) centre (-2.9437, -10.1302) ccw
  arc A12 (-2.6646, -9.1699) -> (-2.2773, -9.2737) centre (0, 0) ccw
  arc A13 (-1.5263, -10.3893) -> (-2.2773, -9.2737) centre (-2.5158, -10.2448) ccw
  line L6 (-1.5263, -10.3893) -> (-1.6383, -11.1567)
  spline S6 degree 5 poles (-1.6383, -11.1567) (-1.6395, -11.1647) (-1.6416, -11.1807) (-1.6439, -11.2048) (-1.6456, -11.237) (-1.6458, -11.2774) (-1.6445, -11.318) (-1.6423, -11.3587) (-1.6396, -11.3994) (-1.6366, -11.4401) (-1.6333, -11.4809) (-1.6295, -11.5218) (-1.625, -11.5626) (-1.6199, -11.6035) (-1.614, -11.6445) (-1.6075, -11.6854) (-1.6005, -11.7264) (-1.5929, -11.7674) (-1.585, -11.8084) (-1.5766, -11.8494) (-1.5678, -11.8905) (-1.5587, -11.9315) (-1.5491, -11.9725) (-1.539, -12.0135) (-1.5285, -12.0545) (-1.5175, -12.0956) (-1.5062, -12.1366) (-1.4944, -12.1776) (-1.4823, -12.2186) (-1.4698, -12.2595) (-1.4569, -12.3005) (-1.4437, -12.3414) (-1.4301, -12.3824) (-1.4161, -12.4233) (-1.4018, -12.4641) (-1.3871, -12.505) (-1.372, -12.5458) (-1.3566, -12.5866) (-1.3409, -12.6274) (-1.3248, -12.6681) (-1.3084, -12.7088) (-1.2917, -12.7495) (-1.2746, -12.7902) (-1.2572, -12.8308) (-1.2395, -12.8713) (-1.2215, -12.9119) (-1.2031, -12.9523) (-1.1844, -12.9928) (-1.1654, -13.0332) (-1.1461, -13.0735) (-1.1265, -13.1138) (-1.1066, -13.1541) (-1.0863, -13.1943) (-1.0658, -13.2345) (-1.045, -13.2746) (-1.0239, -13.3146) (-1.0024, -13.3546) (-0.9807, -13.3946) (-0.9587, -13.4344) (-0.9364, -13.4743) (-0.9138, -13.514) (-0.8909, -13.5538) (-0.8678, -13.5934) (-0.8443, -13.633) (-0.8206, -13.6725) (-0.7966, -13.712) (-0.7723, -13.7514) (-0.7477, -13.7907) (-0.7229, -13.8299) (-0.6978, -13.8691) (-0.6724, -13.9082) (-0.6518, -13.9395) (-0.6363, -13.9629) (-0.6259, -13.9784) (-0.6207, -13.9862) knots 0 0 0 0 0 0 0.01428571 0.02857143 0.04285714 0.05714286 0.07142857 0.08571429 0.1 0.11428571 0.12857143 0.14285714 0.15714286 0.17142857 0.18571429 0.2 0.21428571 0.22857143 0.24285714 0.25714286 0.27142857 0.28571429 0.3 0.31428571 0.32857143 0.34285714 0.35714286 0.37142857 0.38571429 0.4 0.41428571 0.42857143 0.44285714 0.45714286 0.47142857 0.48571429 0.5 0.51428571 0.52857143 0.54285714 0.55714286 0.57142857 0.58571429 0.6 0.61428571 0.62857143 0.64285714 0.65714286 0.67142857 0.68571429 0.7 0.71428571 0.72857143 0.74285714 0.75714286 0.77142857 0.78571429 0.8 0.81428571 0.82857143 0.84285714 0.85714286 0.87142857 0.88571429 0.9 0.91428571 0.92857143 0.94285714 0.95714286 0.97142857 0.98571429 1 1 1 1 1 1
  arc A14 (-0.6207, -13.9862) -> (0.6207, -13.9862) centre (0, 0) ccw
  spline S7 degree 5 poles (0.6207, -13.9862) (0.6259, -13.9784) (0.6363, -13.9629) (0.6518, -13.9395) (0.6724, -13.9082) (0.6978, -13.8691) (0.7229, -13.8299) (0.7477, -13.7907) (0.7723, -13.7514) (0.7966, -13.712) (0.8206, -13.6725) (0.8443, -13.633) (0.8678, -13.5934) (0.8909, -13.5538) (0.9138, -13.514) (0.9364, -13.4743) (0.9587, -13.4344) (0.9807, -13.3946) (1.0024, -13.3546) (1.0239, -13.3146) (1.045, -13.2746) (1.0658, -13.2345) (1.0863, -13.1943) (1.1066, -13.1541) (1.1265, -13.1138) (1.1461, -13.0735) (1.1654, -13.0332) (1.1844, -12.9928) (1.2031, -12.9523) (1.2215, -12.9119) (1.2395, -12.8713) (1.2572, -12.8308) (1.2746, -12.7902) (1.2917, -12.7495) (1.3084, -12.7088) (1.3248, -12.6681) (1.3409, -12.6274) (1.3566, -12.5866) (1.372, -12.5458) (1.3871, -12.505) (1.4018, -12.4641) (1.4161, -12.4233) (1.4301, -12.3824) (1.4437, -12.3414) (1.4569, -12.3005) (1.4698, -12.2595) (1.4823, -12.2186) (1.4944, -12.1776) (1.5062, -12.1366) (1.5175, -12.0956) (1.5285, -12.0545) (1.539, -12.0135) (1.5491, -11.9725) (1.5587, -11.9315) (1.5678, -11.8905) (1.5766, -11.8494) (1.585, -11.8084) (1.5929, -11.7674) (1.6005, -11.7264) (1.6075, -11.6854) (1.614, -11.6445) (1.6199, -11.6035) (1.625, -11.5626) (1.6295, -11.5218) (1.6333, -11.4809) (1.6366, -11.4401) (1.6396, -11.3994) (1.6423, -11.3587) (1.6445, -11.318) (1.6458, -11.2774) (1.6456, -11.237) (1.6439, -11.2048) (1.6416, -11.1807) (1.6395, -11.1647) (1.6383, -11.1567) knots -1 -1 -1 -1 -1 -1 -0.98571429 -0.97142857 -0.95714286 -0.94285714 -0.92857143 -0.91428571 -0.9 -0.88571429 -0.87142857 -0.85714286 -0.84285714 -0.82857143 -0.81428571 -0.8 -0.78571429 -0.77142857 -0.75714286 -0.74285714 -0.72857143 -0.71428571 -0.7 -0.68571429 -0.67142857 -0.65714286 -0.64285714 -0.62857143 -0.61428571 -0.6 -0.58571429 -0.57142857 -0.55714286 -0.54285714 -0.52857143 -0.51428571 -0.5 -0.48571429 -0.47142857 -0.45714286 -0.44285714 -0.42857143 -0.41428571 -0.4 -0.38571429 -0.37142857 -0.35714286 -0.34285714 -0.32857143 -0.31428571 -0.3 -0.28571429 -0.27142857 -0.25714286 -0.24285714 -0.22857143 -0.21428571 -0.2 -0.18571429 -0.17142857 -0.15714286 -0.14285714 -0.12857143 -0.11428571 -0.1 -0.08571429 -0.07142857 -0.05714286 -0.04285714 -0.02857143 -0.01428571 0 0 0 0 0 0
  line L7 (1.6383, -11.1567) -> (1.5263, -10.3893)
  arc A15 (2.2773, -9.2737) -> (1.5263, -10.3893) centre (2.5158, -10.2448) ccw
  arc A16 (2.2773, -9.2737) -> (2.6646, -9.1699) centre (0, 0) ccw
  arc A17 (3.8729, -9.7605) -> (2.6646, -9.1699) centre (2.9437, -10.1302) ccw
  line L8 (3.8729, -9.7605) -> (4.1595, -10.4811)
  spline S8 degree 5 poles (4.1595, -10.4811) (4.1625, -10.4886) (4.1687, -10.5035) (4.1787, -10.5256) (4.1933, -10.5543) (4.2134, -10.5894) (4.2349, -10.6239) (4.2571, -10.658) (4.2797, -10.692) (4.3027, -10.7258) (4.326, -10.7594) (4.3497, -10.7929) (4.374, -10.826) (4.3989, -10.8589) (4.4244, -10.8914) (4.4505, -10.9236) (4.4772, -10.9556) (4.5042, -10.9873) (4.5316, -11.0189) (4.5593, -11.0502) (4.5874, -11.0814) (4.6159, -11.1123) (4.6447, -11.143) (4.674, -11.1735) (4.7036, -11.2038) (4.7336, -11.2338) (4.7639, -11.2637) (4.7946, -11.2933) (4.8256, -11.3227) (4.8569, -11.352) (4.8885, -11.381) (4.9204, -11.4099) (4.9527, -11.4385) (4.9852, -11.4669) (5.0181, -11.4952) (5.0512, -11.5232) (5.0847, -11.551) (5.1184, -11.5787) (5.1524, -11.6061) (5.1867, -11.6334) (5.2213, -11.6604) (5.2561, -11.6873) (5.2912, -11.7139) (5.3266, -11.7404) (5.3622, -11.7666) (5.3981, -11.7927) (5.4343, -11.8186) (5.4707, -11.8443) (5.5073, -11.8698) (5.5442, -11.8951) (5.5813, -11.9202) (5.6187, -11.9451) (5.6563, -11.9698) (5.6942, -11.9943) (5.7323, -12.0186) (5.7706, -12.0427) (5.8092, -12.0667) (5.848, -12.0904) (5.887, -12.1139) (5.9262, -12.1373) (5.9656, -12.1604) (6.0053, -12.1834) (6.0452, -12.2061) (6.0853, -12.2287) (6.1256, -12.251) (6.1661, -12.2732) (6.2069, -12.2952) (6.2478, -12.3169) (6.2889, -12.3385) (6.3303, -12.3599) (6.3718, -12.3811) (6.4052, -12.3979) (6.4304, -12.4104) (6.4472, -12.4186) (6.4556, -12.4228) knots 0 0 0 0 0 0 0.01428571 0.02857143 0.04285714 0.05714286 0.07142857 0.08571429 0.1 0.11428571 0.12857143 0.14285714 0.15714286 0.17142857 0.18571429 0.2 0.21428571 0.22857143 0.24285714 0.25714286 0.27142857 0.28571429 0.3 0.31428571 0.32857143 0.34285714 0.35714286 0.37142857 0.38571429 0.4 0.41428571 0.42857143 0.44285714 0.45714286 0.47142857 0.48571429 0.5 0.51428571 0.52857143 0.54285714 0.55714286 0.57142857 0.58571429 0.6 0.61428571 0.62857143 0.64285714 0.65714286 0.67142857 0.68571429 0.7 0.71428571 0.72857143 0.74285714 0.75714286 0.77142857 0.78571429 0.8 0.81428571 0.82857143 0.84285714 0.85714286 0.87142857 0.88571429 0.9 0.91428571 0.92857143 0.94285714 0.95714286 0.97142857 0.98571429 1 1 1 1 1 1
  arc A18 (6.4556, -12.4228) -> (7.5307, -11.8021) centre (0, 0) ccw
  spline S9 degree 5 poles (7.5307, -11.8021) (7.5313, -11.7927) (7.5325, -11.774) (7.5342, -11.746) (7.5364, -11.7087) (7.5388, -11.6621) (7.541, -11.6156) (7.5429, -11.5692) (7.5445, -11.5229) (7.5458, -11.4766) (7.5469, -11.4305) (7.5477, -11.3844) (7.5482, -11.3384) (7.5484, -11.2924) (7.5484, -11.2466) (7.5481, -11.2009) (7.5475, -11.1552) (7.5466, -11.1097) (7.5454, -11.0642) (7.544, -11.0189) (7.5423, -10.9736) (7.5403, -10.9285) (7.538, -10.8834) (7.5354, -10.8385) (7.5325, -10.7937) (7.5293, -10.7489) (7.5259, -10.7044) (7.5221, -10.6599) (7.5181, -10.6155) (7.5137, -10.5713) (7.5091, -10.5271) (7.5042, -10.4832) (7.4989, -10.4393) (7.4934, -10.3956) (7.4876, -10.352) (7.4814, -10.3085) (7.475, -10.2652) (7.4682, -10.222) (7.4611, -10.179) (7.4538, -10.1361) (7.4461, -10.0934) (7.438, -10.0508) (7.4297, -10.0084) (7.421, -9.9662) (7.412, -9.9241) (7.4027, -9.8822) (7.393, -9.8404) (7.383, -9.7989) (7.3727, -9.7575) (7.362, -9.7163) (7.351, -9.6753) (7.3396, -9.6345) (7.3278, -9.594) (7.3156, -9.5536) (7.303, -9.5135) (7.2901, -9.4736) (7.2768, -9.4339) (7.2632, -9.3944) (7.2492, -9.3551) (7.2349, -9.3161) (7.22, -9.2774) (7.2046, -9.239) (7.1886, -9.201) (7.172, -9.1634) (7.1549, -9.1261) (7.1374, -9.0891) (7.1196, -9.0523) (7.1016, -9.0157) (7.0831, -8.9794) (7.064, -8.9437) (7.0436, -8.9087) (7.0261, -8.8816) (7.012, -8.862) (7.0022, -8.8491) (6.9972, -8.8428) knots -1 -1 -1 -1 -1 -1 -0.98571429 -0.97142857 -0.95714286 -0.94285714 -0.92857143 -0.91428571 -0.9 -0.88571429 -0.87142857 -0.85714286 -0.84285714 -0.82857143 -0.81428571 -0.8 -0.78571429 -0.77142857 -0.75714286 -0.74285714 -0.72857143 -0.71428571 -0.7 -0.68571429 -0.67142857 -0.65714286 -0.64285714 -0.62857143 -0.61428571 -0.6 -0.58571429 -0.57142857 -0.55714286 -0.54285714 -0.52857143 -0.51428571 -0.5 -0.48571429 -0.47142857 -0.45714286 -0.44285714 -0.42857143 -0.41428571 -0.4 -0.38571429 -0.37142857 -0.35714286 -0.34285714 -0.32857143 -0.31428571 -0.3 -0.28571429 -0.27142857 -0.25714286 -0.24285714 -0.22857143 -0.21428571 -0.2 -0.18571429 -0.17142857 -0.15714286 -0.14285714 -0.12857143 -0.11428571 -0.1 -0.08571429 -0.07142857 -0.05714286 -0.04285714 -0.02857143 -0.01428571 0 0 0 0 0 0
  line L9 (6.9972, -8.8428) -> (6.5164, -8.2343)
  arc A19 (6.609, -6.8926) -> (6.5164, -8.2343) centre (7.3011, -7.6144) ccw
  arc A20 (6.609, -6.8926) -> (6.8926, -6.609) centre (0, 0) ccw
  arc A21 (8.2343, -6.5164) -> (6.8926, -6.609) centre (7.6144, -7.3011) ccw
  line L10 (8.2343, -6.5164) -> (8.8428, -6.9972)
  spline S10 degree 5 poles (8.8428, -6.9972) (8.8491, -7.0022) (8.862, -7.012) (8.8816, -7.0261) (8.9087, -7.0436) (8.9437, -7.064) (8.9794, -7.0831) (9.0157, -7.1016) (9.0523, -7.1196) (9.0891, -7.1374) (9.1261, -7.1549) (9.1634, -7.172) (9.201, -7.1886) (9.239, -7.2046) (9.2774, -7.22) (9.3161, -7.2349) (9.3551, -7.2492) (9.3944, -7.2632) (9.4339, -7.2768) (9.4736, -7.2901) (9.5135, -7.303) (9.5536, -7.3156) (9.594, -7.3278) (9.6345, -7.3396) (9.6753, -7.351) (9.7163, -7.362) (9.7575, -7.3727) (9.7989, -7.383) (9.8404, -7.393) (9.8822, -7.4027) (9.9241, -7.412) (9.9662, -7.421) (10.0084, -7.4297) (10.0508, -7.438) (10.0934, -7.4461) (10.1361, -7.4538) (10.179, -7.4611) (10.222, -7.4682) (10.2652, -7.475) (10.3085, -7.4814) (10.352, -7.4876) (10.3956, -7.4934) (10.4393, -7.4989) (10.4832, -7.5042) (10.5271, -7.5091) (10.5713, -7.5137) (10.6155, -7.5181) (10.6599, -7.5221) (10.7044, -7.5259) (10.7489, -7.5293) (10.7937, -7.5325) (10.8385, -7.5354) (10.8834, -7.538) (10.9285, -7.5403) (10.9736, -7.5423) (11.0189, -7.544) (11.0642, -7.5454) (11.1097, -7.5466) (11.1552, -7.5475) (11.2009, -7.5481) (11.2466, -7.5484) (11.2924, -7.5484) (11.3384, -7.5482) (11.3844, -7.5477) (11.4305, -7.5469) (11.4766, -7.5458) (11.5229, -7.5445) (11.5692, -7.5429) (11.6156, -7.541) (11.6621, -7.5388) (11.7087, -7.5364) (11.746, -7.5342) (11.774, -7.5325) (11.7927, -7.5313) (11.8021, -7.5307) knots 0 0 0 0 0 0 0.01428571 0.02857143 0.04285714 0.05714286 0.07142857 0.08571429 0.1 0.11428571 0.12857143 0.14285714 0.15714286 0.17142857 0.18571429 0.2 0.21428571 0.22857143 0.24285714 0.25714286 0.27142857 0.28571429 0.3 0.31428571 0.32857143 0.34285714 0.35714286 0.37142857 0.38571429 0.4 0.41428571 0.42857143 0.44285714 0.45714286 0.47142857 0.48571429 0.5 0.51428571 0.52857143 0.54285714 0.55714286 0.57142857 0.58571429 0.6 0.61428571 0.62857143 0.64285714 0.65714286 0.67142857 0.68571429 0.7 0.71428571 0.72857143 0.74285714 0.75714286 0.77142857 0.78571429 0.8 0.81428571 0.82857143 0.84285714 0.85714286 0.87142857 0.88571429 0.9 0.91428571 0.92857143 0.94285714 0.95714286 0.97142857 0.98571429 1 1 1 1 1 1
  arc A22 (11.8021, -7.5307) -> (12.4228, -6.4556) centre (0, 0) ccw
  spline S11 degree 5 poles (12.4228, -6.4556) (12.4186, -6.4472) (12.4104, -6.4304) (12.3979, -6.4052) (12.3811, -6.3718) (12.3599, -6.3303) (12.3385, -6.2889) (12.3169, -6.2478) (12.2952, -6.2069) (12.2732, -6.1661) (12.251, -6.1256) (12.2287, -6.0853) (12.2061, -6.0452) (12.1834, -6.0053) (12.1604, -5.9656) (12.1373, -5.9262) (12.1139, -5.887) (12.0904, -5.848) (12.0667, -5.8092) (12.0427, -5.7706) (12.0186, -5.7323) (11.9943, -5.6942) (11.9698, -5.6563) (11.9451, -5.6187) (11.9202, -5.5813) (11.8951, -5.5442) (11.8698, -5.5073) (11.8443, -5.4707) (11.8186, -5.4343) (11.7927, -5.3981) (11.7666, -5.3622) (11.7404, -5.3266) (11.7139, -5.2912) (11.6873, -5.2561) (11.6604, -5.2213) (11.6334, -5.1867) (11.6061, -5.1524) (11.5787, -5.1184) (11.551, -5.0847) (11.5232, -5.0512) (11.4952, -5.0181) (11.4669, -4.9852) (11.4385, -4.9527) (11.4099, -4.9204) (11.381, -4.8885) (11.352, -4.8569) (11.3227, -4.8256) (11.2933, -4.7946) (11.2637, -4.7639) (11.2338, -4.7336) (11.2038, -4.7036) (11.1735, -4.674) (11.143, -4.6447) (11.1123, -4.6159) (11.0814, -4.5874) (11.0502, -4.5593) (11.0189, -4.5316) (10.9873, -4.5042) (10.9556, -4.4772) (10.9236, -4.4505) (10.8914, -4.4244) (10.8589, -4.3989) (10.826, -4.374) (10.7929, -4.3497) (10.7594, -4.326) (10.7258, -4.3027) (10.692, -4.2797) (10.658, -4.2571) (10.6239, -4.2349) (10.5894, -4.2134) (10.5543, -4.1933) (10.5256, -4.1787) (10.5035, -4.1687) (10.4886, -4.1625) (10.4811, -4.1595) knots -1 -1 -1 -1 -1 -1 -0.98571429 -0.97142857 -0.95714286 -0.94285714 -0.92857143 -0.91428571 -0.9 -0.88571429 -0.87142857 -0.85714286 -0.84285714 -0.82857143 -0.81428571 -0.8 -0.78571429 -0.77142857 -0.75714286 -0.74285714 -0.72857143 -0.71428571 -0.7 -0.68571429 -0.67142857 -0.65714286 -0.64285714 -0.62857143 -0.61428571 -0.6 -0.58571429 -0.57142857 -0.55714286 -0.54285714 -0.52857143 -0.51428571 -0.5 -0.48571429 -0.47142857 -0.45714286 -0.44285714 -0.42857143 -0.41428571 -0.4 -0.38571429 -0.37142857 -0.35714286 -0.34285714 -0.32857143 -0.31428571 -0.3 -0.28571429 -0.27142857 -0.25714286 -0.24285714 -0.22857143 -0.21428571 -0.2 -0.18571429 -0.17142857 -0.15714286 -0.14285714 -0.12857143 -0.11428571 -0.1 -0.08571429 -0.07142857 -0.05714286 -0.04285714 -0.02857143 -0.01428571 0 0 0 0 0 0
  line L11 (10.4811, -4.1595) -> (9.7605, -3.8729)
  arc A23 (9.1699, -2.6646) -> (9.7605, -3.8729) centre (10.1302, -2.9437) ccw
  arc A24 (9.1699, -2.6646) -> (9.2737, -2.2773) centre (0, 0) ccw
  arc A25 (10.3893, -1.5263) -> (9.2737, -2.2773) centre (10.2448, -2.5158) ccw
  line L12 (10.3893, -1.5263) -> (11.1567, -1.6383)
  spline S12 degree 5 poles (11.1567, -1.6383) (11.1647, -1.6395) (11.1807, -1.6416) (11.2048, -1.6439) (11.237, -1.6456) (11.2774, -1.6458) (11.318, -1.6445) (11.3587, -1.6423) (11.3994, -1.6396) (11.4401, -1.6366) (11.4809, -1.6333) (11.5218, -1.6295) (11.5626, -1.625) (11.6035, -1.6199) (11.6445, -1.614) (11.6854, -1.6075) (11.7264, -1.6005) (11.7674, -1.5929) (11.8084, -1.585) (11.8494, -1.5766) (11.8905, -1.5678) (11.9315, -1.5587) (11.9725, -1.5491) (12.0135, -1.539) (12.0545, -1.5285) (12.0956, -1.5175) (12.1366, -1.5062) (12.1776, -1.4944) (12.2186, -1.4823) (12.2595, -1.4698) (12.3005, -1.4569) (12.3414, -1.4437) (12.3824, -1.4301) (12.4233, -1.4161) (12.4641, -1.4018) (12.505, -1.3871) (12.5458, -1.372) (12.5866, -1.3566) (12.6274, -1.3409) (12.6681, -1.3248) (12.7088, -1.3084) (12.7495, -1.2917) (12.7902, -1.2746) (12.8308, -1.2572) (12.8713, -1.2395) (12.9119, -1.2215) (12.9523, -1.2031) (12.9928, -1.1844) (13.0332, -1.1654) (13.0735, -1.1461) (13.1138, -1.1265) (13.1541, -1.1066) (13.1943, -1.0863) (13.2345, -1.0658) (13.2746, -1.045) (13.3146, -1.0239) (13.3546, -1.0024) (13.3946, -0.9807) (13.4344, -0.9587) (13.4743, -0.9364) (13.514, -0.9138) (13.5538, -0.8909) (13.5934, -0.8678) (13.633, -0.8443) (13.6725, -0.8206) (13.712, -0.7966) (13.7514, -0.7723) (13.7907, -0.7477) (13.8299, -0.7229) (13.8691, -0.6978) (13.9082, -0.6724) (13.9395, -0.6518) (13.9629, -0.6363) (13.9784, -0.6259) (13.9862, -0.6207) knots 0 0 0 0 0 0 0.01428571 0.02857143 0.04285714 0.05714286 0.07142857 0.08571429 0.1 0.11428571 0.12857143 0.14285714 0.15714286 0.17142857 0.18571429 0.2 0.21428571 0.22857143 0.24285714 0.25714286 0.27142857 0.28571429 0.3 0.31428571 0.32857143 0.34285714 0.35714286 0.37142857 0.38571429 0.4 0.41428571 0.42857143 0.44285714 0.45714286 0.47142857 0.48571429 0.5 0.51428571 0.52857143 0.54285714 0.55714286 0.57142857 0.58571429 0.6 0.61428571 0.62857143 0.64285714 0.65714286 0.67142857 0.68571429 0.7 0.71428571 0.72857143 0.74285714 0.75714286 0.77142857 0.78571429 0.8 0.81428571 0.82857143 0.84285714 0.85714286 0.87142857 0.88571429 0.9 0.91428571 0.92857143 0.94285714 0.95714286 0.97142857 0.98571429 1 1 1 1 1 1
  arc A26 (13.9862, -0.6207) -> (13.9862, 0.6207) centre (0, 0) ccw